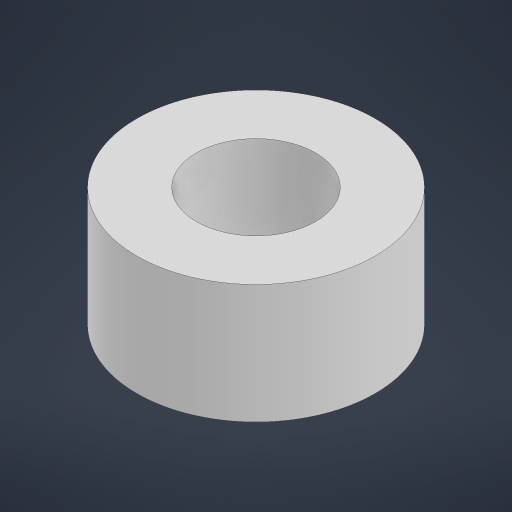
# Autodesk Inventor part: base
Saved by Autodesk Inventor 2024.3 (Build 283343000, 343)
## iProperties
Created: 2024-09-28
Part Number: base
Material: Generic
Document SubType Name: Modeling
Designer: sam
Density: 1 g/cm^3
Appearance: Default
Sheet Metal Rule: Default
Author: sam
Autodesk Inventor part; units mm, degrees
ref_plane "YZ Plane" through (0, 0, 0) normal (1, 0, 0) x (0, 1, 0)
ref_plane "XZ Plane" through (0, 0, 0) normal (0, 1, 0) x (-1, 0, 0)
ref_plane "XY Plane" through (0, 0, 0) normal (0, 0, 1) x (1, 0, 0)
sketch "Sketch1" plane through (0, 0, 0) normal (0, 1, 0) x (-1, 0, 0)
  line L0 (0, -5) -> (0, -5)
  line L1 (5, 0) -> (5, 0)
  line L2 (0, 5) -> (0, 5)
  line L3 (-5, 0) -> (-5, 0)
  line L4 (-5, -5) -> (5, 5) construction
  line L5 (5, -5) -> (-5, 5) construction
  circle A0 centre (0, 0) radius 2.5
  arc A1 (0, 5) -> (-5, 0) centre (0, 0) ccw
  arc A2 (5, 0) -> (0, 5) centre (0, 0) ccw
  arc A3 (0, -5) -> (5, 0) centre (0, 0) ccw
  arc A4 (-5, 0) -> (0, -5) centre (0, 0) ccw
  point P0 (0, 5)
  point P1 (-5, 0)
  dimension "d0" = 10
  dimension "d1" = 10
  dimension "d46" = 5
  dimension "d47" = 5
  constraints: 12 end point, 8 point on circle, 8 point on line, 8 tangent, 5 centre point, 3 concentric, 2 midpoint, 2 parallel, 1 coincident, 1 horizontal, 1 perpendicular
  measures "d0" distance of L5.end L4.end
  measures "d1" distance of L4.end L5.start
  measures "d46" diameter of A0
  measures "d47" radius of A1
extrude "Extrusion1" add sketch "Sketch1" along normal blind 5
equation "\"BendRadius\" = Thickness"
equation "\"BendReliefWidth\" = Thickness"
equation "\"BendReliefDepth\" = 0.5 * Thickness"
equation "\"CornerReliefSize\" = 4 * Thickness"
equation "\"MinimumRemnant\" = 2 * Thickness"
equation "\"TransitionRadius\" = BendRadius"
equation "\"JacobiRadiusSize\" = BendRadius"
equation "\"GapSize\" = Thickness"
equation "\"Thickness\" = 3.048"
body "Solid1"
